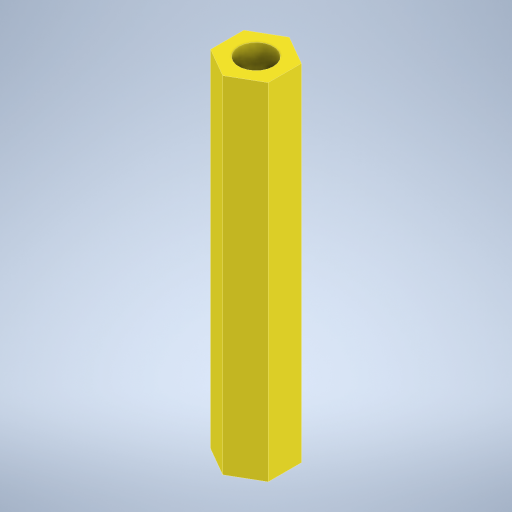
# Autodesk Inventor part: Varrilla_Cobre
Saved by Autodesk Inventor 2023 (Build 270158000, 158)
## iProperties
Created: 2024-08-05
Part Number: Varrilla_Cobre
Material: Generic
Document SubType Name: Modeling
Designer: LEGION
Density: 1 g/cm^3
Appearance: Default
Author: LEGION
Autodesk Inventor part; units mm, degrees
ref_plane "YZ Plane" through (0, 0, 0) normal (1, 0, 0) x (0, 1, 0)
ref_plane "XZ Plane" through (0, 0, 0) normal (0, 1, 0) x (-1, 0, 0)
ref_plane "XY Plane" through (0, 0, 0) normal (0, 0, 1) x (1, 0, 0)
sketch "Sketch1" plane through (0, 0, 0) normal (0, 1, 0) x (-1, 0, 0)
  circle A0 centre (0, 0) radius 1.5
  line L0 (-2.5, -1.4434) -> (-2.5, 1.4434)
  line L1 (-2.5, 1.4434) -> (0, 2.8868)
  line L2 (0, 2.8868) -> (2.5, 1.4434)
  line L3 (2.5, 1.4434) -> (2.5, -1.4434)
  line L4 (2.5, -1.4434) -> (0, -2.8868)
  line L5 (0, -2.8868) -> (-2.5, -1.4434)
  point P0 (-2.5, 0)
  dimension "d0" = 3
  dimension "d1" = 5
  constraints: 12 end point, 2 coincident, 1 centre point, 1 midpoint, 1 vertical, 13 other
  measures "d0" diameter of A0
  measures "d1" distance from line of point (-2.5, 0) L3
extrude "Extrusion1" add sketch "Sketch1" along normal blind 30
body "Solid1"
